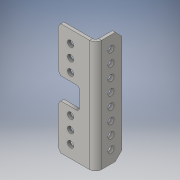
# Autodesk Inventor part: Transmission bracket
Saved by Autodesk Inventor 2016 SP2 (Build 200236200, 236)
## iProperties
Created: 2018-01-18
Part Number: Transmission bracket
Material: Generic
Document SubType Name: Sheet Metal
Designer: CAD
Density: 1 g/cm^3
Sheet Metal Rule: Default
Appearance: Default
Author: CAD
Autodesk Inventor part; units mm, degrees
ref_plane "YZ Plane" through (0, 0, 0) normal (1, 0, 0) x (0, 1, 0)
ref_plane "XZ Plane" through (0, 0, 0) normal (0, 1, 0) x (-1, 0, 0)
ref_plane "XY Plane" through (0, 0, 0) normal (0, 0, 1) x (1, 0, 0)
sketch "Sketch1" plane through (0, 0, 0) normal (0, 0, 1) x (1, 0, 0)
  line L0 (0, 46.0375) -> (-2.644, 42.0764)
  line L1 (-2.644, 42.0764) -> (-2.644, 3.9764)
  line L2 (-2.644, 3.9764) -> (0, 0)
  line L3 (0, 46.0375) -> (19.05, 46.0375)
  line L4 (19.05, 46.0375) -> (19.05, 68.2625)
  line L5 (19.05, 57.15) -> (14.1908, 57.15)
  line L6 (0, 68.2625) -> (-2.644, 72.2236)
  line L7 (-2.644, 72.2236) -> (-2.644, 110.3236)
  line L8 (-2.644, 110.3236) -> (0, 114.3)
  line L9 (0, 68.2625) -> (19.05, 68.2625)
  line L10 (19.05, 68.2625) -> (19.05, 46.0375)
  line L11 (35.456, 114.3) -> (0, 114.3)
  line L12 (35.456, 114.3) -> (35.456, 0)
  line L13 (0, 0) -> (35.456, 0)
  line L14 (218.3648, 132.2525) -> (215.7208, 128.2914)
  line L15 (215.7208, 128.2914) -> (215.7208, 90.1914)
  line L16 (215.7208, 90.1914) -> (218.3648, 86.215)
  line L17 (218.3648, 132.2525) -> (234.2398, 132.2525)
  line L18 (218.3648, 154.4775) -> (215.7208, 158.4387)
  line L19 (215.7208, 158.4387) -> (215.7208, 196.5387)
  line L20 (215.7208, 196.5387) -> (218.3648, 200.515)
  line L21 (218.3648, 154.4775) -> (234.2398, 154.4775)
  line L22 (253.8208, 200.515) -> (218.3648, 200.515)
  line L23 (253.8208, 200.515) -> (253.8208, 86.215)
  line L24 (218.3648, 86.215) -> (253.8208, 86.215)
  line L25 (379.0105, 160.3375) -> (376.3665, 156.3764)
  line L26 (376.3665, 156.3764) -> (376.3665, 118.2764)
  line L27 (376.3665, 118.2764) -> (379.0105, 114.3)
  line L28 (379.0105, 160.3375) -> (398.0605, 160.3375)
  line L29 (398.0605, 160.3375) -> (398.0605, 182.5625)
  line L30 (398.0605, 171.45) -> (393.2013, 171.45)
  line L31 (379.0105, 182.5625) -> (376.3665, 186.5236)
  line L32 (376.3665, 186.5236) -> (376.3665, 224.6236)
  line L33 (376.3665, 224.6236) -> (379.0105, 228.6)
  line L34 (379.0105, 182.5625) -> (398.0605, 182.5625)
  line L35 (398.0605, 182.5625) -> (398.0605, 160.3375)
  line L36 (414.4665, 228.6) -> (379.0105, 228.6)
  line L37 (414.4665, 228.6) -> (414.4665, 114.3)
  line L38 (379.0105, 114.3) -> (414.4665, 114.3)
  line L39 (237.4148, 151.3025) -> (237.4148, 135.4275)
  arc A0 (237.4148, 151.3025) -> (234.2398, 154.4775) centre (234.2398, 151.3025) ccw
  arc A1 (234.2398, 132.2525) -> (237.4148, 135.4275) centre (234.2398, 135.4275) ccw
  dimension "d1" = 46.0375
  dimension "d5" = 38.1
  dimension "d6" = 4.7625
  dimension "d8" = 4.7752
  dimension "d9" = 19.05
  dimension "d12" = 22.225
  dimension "d14" = 114.3
  dimension "d15" = 16.406
  dimension "d16" = 21.2652
  dimension "d26" = 46.0375
  dimension "d27" = 38.1
  dimension "d28" = 4.7625
  dimension "d29" = 4.7752
  dimension "d30" = 19.05
  dimension "d31" = 22.225
  dimension "d32" = 114.3
  dimension "d33" = 16.406
  dimension "d34" = 21.2652
  dimension "d35" = 3.175
  measures "d1" distance of L2.end L0.start
  measures "d5" distance of L0.end L1.end
  measures "d6" distance of L0.start L0.end
  measures "d8" distance of L1.end L2.end
  measures "d9" distance of L0.start L3.end
  measures "d12" distance of L3.end L4.end
  measures "d14" distance of L11.start L12.end
  measures "d15" distance between parallel lines of L12 L4
  measures "d16" distance from line of L5.end L12
  measures "d26" distance of L38.start L28.start
  measures "d27" distance of L25.end L26.end
  measures "d28" distance of L28.start L25.end
  measures "d29" distance of L26.end L38.start
  measures "d30" distance of L28.start L29.start
  measures "d31" distance of L29.start L29.end
  measures "d32" distance of L37.start L37.end
  measures "d33" distance between parallel lines of L37 L29
  measures "d34" distance from line of L30.end L37
  measures "d35" radius of A0
extrude "Plate1" add sketch "Sketch1" along normal blind 3.048 contours L17 A1 L39 A0 L21 L18 L19 L20 L22 L23 L24 L16 L15 L14
sketch "Sketch2" plane through (253.8208, 86.215, 0) normal (1, 0, 0) x (0, 0, -1)
  line L0 (0, 114.3) -> (17.0773, 114.3)
  line L1 (23.8125, 107.5648) -> (23.8125, 6.7352)
  line L2 (0, 0) -> (0, 114.3)
  line L3 (0, 0) -> (17.0773, 0)
  line L4 (0, 0) -> (0, 114.3)
  line L5 (17.0773, 114.3) -> (23.8125, 107.5648)
  line L6 (23.8125, 57.15) -> (19.0341, 57.15)
  line L7 (17.0773, 0) -> (23.8125, 6.7352)
  point P0 (0, -86.215)
  dimension "d38" = 45
  dimension "d39" = 9.525
  measures "d38" angle of L0 L5
  measures "d39" distance of L0.end L1.start
sheet face with bend "Face2" sketch "Sketch2" thickness 3.048 toward (-1, 0, 0) bend radius 3.048 relief straight relief width 3.048 relief depth 1.524
bend "Bend1"
sketch "Sketch3" plane through (0, 0, 0) normal (0, 0, -1) x (-1, 0, 0)
  line L0 (-218.3648, 154.4775) -> (-234.2398, 154.4775) projected
  line L1 (-215.7208, 196.5387) -> (-215.7208, 158.4387) projected
  line L2 (-237.4148, 135.4275) -> (-237.4148, 151.3025) projected
  line L3 (-237.4148, 143.365) -> (-228.4208, 143.365)
  point P0 (0, 0)
  point P1 (-228.4208, 162.415)
  point P2 (-228.4208, 175.115)
  point P3 (-228.4208, 187.815)
  point P4 (-228.4208, 124.315)
  point P5 (-228.4208, 111.615)
  point P6 (-228.4208, 98.915)
  dimension "d45" = 7.9375
  dimension "d46" = 12.7
  dimension "d47" = 12.7
  dimension "d48" = 12.7
  dimension "d49" = 12.7
  dimension "d50" = 12.7
  constraints: 3 symmetric about line, 2 end point, 1 horizontal, 1 midpoint
  measures "d45" distance from line of point (-228.421, 162.415) L0
  measures "d46" distance of point (-228.421, 175.115) point (-228.421, 162.415)
  measures "d47" distance of point (-228.421, 187.815) point (-228.421, 175.115)
  measures "d48" distance from line of L1 point (-228.421, 175.115)
  measures "d49" distance from line of L1 point (-228.421, 162.415)
  measures "d50" distance from line of L1 point (-228.421, 187.815)
hole "Hole1" at (228.4208, 162.415, 0) at (228.4208, 175.115, 0) at (228.4208, 187.815, 0) at (228.4208, 98.915, 0) at (228.4208, 111.615, 0) at (228.4208, 124.315, 0) direction (0, 0, 1) diameter 6.35 depth 3.048 tip angle 118
sketch "Sketch4" plane through (253.8208, 86.215, 0) normal (1, 0, 0) x (0, 0, -1)
  line L0 (3.048, 0) -> (17.0773, 0) projected
  line L1 (23.8125, 6.7352) -> (23.8125, 107.5648) projected
  line L2 (23.8125, 107.5648) -> (23.8125, 6.7352)
  point P0 (0, -86.215)
  point P1 (12.7, 12.7)
  point P2 (12.7, 25.4)
  point P3 (12.7, 50.8)
  point P4 (12.7, 63.5)
  point P5 (12.7, 76.2)
  point P6 (12.7, 88.9)
  point P7 (12.7, 101.6)
  point P8 (12.7, 38.1)
  dimension "d58" = 12.7
  dimension "d59" = 12.7
  dimension "d60" = 12.7
  dimension "d61" = 12.7
  dimension "d62" = 12.7
  dimension "d63" = 12.7
  dimension "d64" = 12.7
  dimension "d65" = 12.7
  dimension "d66" = 11.1125
  dimension "d67" = 11.1125
  dimension "d68" = 11.1125
  dimension "d69" = 11.1125
  dimension "d70" = 11.1125
  dimension "d71" = 11.1125
  dimension "d72" = 11.1125
  dimension "d73" = 11.1125
  constraints: 2 end point, 1 collinear
  measures "d58" distance from line of L0 point (12.7, 12.7)
  measures "d59" distance of point (12.7, 25.4) point (12.7, 12.7)
  measures "d60" distance of point (12.7, 38.1) point (12.7, 25.4)
  measures "d61" distance of point (12.7, 50.8) point (12.7, 38.1)
  measures "d62" distance of point (12.7, 63.5) point (12.7, 50.8)
  measures "d63" distance of point (12.7, 76.2) point (12.7, 63.5)
  measures "d64" distance of point (12.7, 88.9) point (12.7, 76.2)
  measures "d65" distance of point (12.7, 101.6) point (12.7, 88.9)
  measures "d66" distance from line of L1 point (12.7, 101.6)
  measures "d67" distance from line of L1 point (12.7, 88.9)
  measures "d68" distance from line of L1 point (12.7, 76.2)
  measures "d69" distance from line of L1 point (12.7, 63.5)
  measures "d70" distance from line of L1 point (12.7, 50.8)
  measures "d71" distance from line of L1 point (12.7, 38.1)
  measures "d72" distance from line of L1 point (12.7, 25.4)
  measures "d73" distance from line of L1 point (12.7, 12.7)
hole "Hole2" at (253.8208, 98.915, -12.7) at (253.8208, 111.615, -12.7) at (253.8208, 137.015, -12.7) at (253.8208, 149.715, -12.7) at (253.8208, 162.415, -12.7) at (253.8208, 175.115, -12.7) at (253.8208, 187.815, -12.7) at (253.8208, 124.315, -12.7) direction (-1, 0, 0) diameter 6.35 depth 3.048 tip angle 118
equation "\"d56\" = Thickness"
equation "\"d79\" = Thickness"
equation "\"d40\" = BendRadius"
equation "\"d41\" = BendReliefWidth"
equation "\"d43\" = MinimumRemnant"
equation "\"d42\" = BendReliefDepth"
equation "\"d44\" = BendRadius"
equation "\"BendRadius\" = Thickness"
equation "\"BendReliefWidth\" = Thickness"
equation "\"BendReliefDepth\" = 0.5 * Thickness"
equation "\"CornerReliefSize\" = 4 * Thickness"
equation "\"MinimumRemnant\" = 2 * Thickness"
equation "\"TransitionRadius\" = BendRadius"
equation "\"JacobiRadiusSize\" = BendRadius"
equation "\"GapSize\" = Thickness"
equation "\"d36\" = BendRadius"
equation "\"Thickness\" = 3.048"
body "Solid1"
